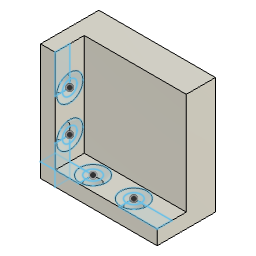
Step3-CornerMagBox-16X (Autodesk Fusion 360 design; units mm, degrees)
Autodesk Fusion 360 part; units mm, degrees
note: some values were not read from the file. Set by a fixed rule: which sketch regions a step uses.
sketch "Sketch1" plane through (0, 0, 0) normal (0, 1, 0) x (1, 0, 0)
  line L0 (0, 0) -> (40, 0)
  line L1 (40, 0) -> (40, -40)
  line L2 (40, -40) -> (0, -40)
  line L3 (0, -40) -> (0, 0)
  dimension "d1" = 40
  dimension "d2" = 40
  constraint horizontal L0
  constraint vertical L1
  constraint horizontal L2
  constraint vertical L3
  constraint coincident L0.start L3.end
  measures "d1" distance of L0.start L0.end
  measures "d2" distance of L0.start L2.end
extrude "Extrude1" add sketch "Sketch1" along normal blind 20
ref_plane "WorkPlane1" through (20, 0, 20) normal (0, -1, 0) x (-1, 0, 0)
sketch "Sketch2" plane through (20, 0, 20) normal (0, -1, 0) x (1, 0, 0)
  line L0 (20, 20) -> (-15, 20)
  line L1 (-15, 20) -> (-15, -15)
  line L2 (-15, -15) -> (20, -15)
  line L3 (20, -15) -> (20, 20)
  dimension "d6" = 35
  dimension "d7" = 35
  constraint horizontal L0
  constraint vertical L1
  constraint horizontal L2
  constraint vertical L3
  measures "d6" distance of L0.start L0.end
  measures "d7" distance of L0.start L2.end
extrude "Extrude2" cut sketch "Sketch2" against normal blind 10
ref_plane "WorkPlane2" through (5, 5, 22.5) normal (1, 0, 0) x (0, 0, -1)
sketch "Sketch3" plane through (5, 5, 22.5) normal (1, 0, 0) x (0, 1, 0)
  circle A0 centre (0, 4.5) radius 2.5
  circle A1 centre (0, -9.5) radius 2.5
  line L0 (-5, 17.5) -> (0, 17.5)
  line L1 (0, 17.5) -> (0, 4.5)
  line L2 (0, 4.5) -> (-5, 4.5)
  line L3 (-5, 4.5) -> (-5, 17.5)
  line L4 (-5, -22.5) -> (0, -22.5)
  line L5 (0, -22.5) -> (0, -9.5)
  line L6 (0, -9.5) -> (-5, -9.5)
  line L7 (-5, -9.5) -> (-5, -22.5)
  circle A2 centre (0, 4.5) radius 4.5
  circle A3 centre (0, -9.5) radius 4.5
  dimension "d11" = 5
  dimension "d12" = 5
  dimension "d35" = 5
  dimension "d36" = 13
  dimension "d37" = 5
  dimension "d38" = 13
  dimension "d39" = 9
  dimension "d40" = 9
  constraint horizontal L0
  constraint vertical L1
  constraint horizontal L2
  constraint vertical L3
  constraint horizontal L4
  constraint vertical L5
  constraint horizontal L6
  constraint vertical L7
  constraint coincident A0.centre L1.end
  constraint coincident A1.centre L5.end
  constraint concentric A0 A2
  constraint concentric A1 A3
  measures "d11" diameter of A0
  measures "d12" diameter of A1
  measures "d35" distance of L0.start L0.end
  measures "d36" distance of L0.start L2.end
  measures "d37" distance of L4.start L4.end
  measures "d38" distance of L4.start L6.end
  measures "d39" diameter of A2
  measures "d40" diameter of A3
extrude "Extrude7" cut sketch "Sketch3" against normal blind 2.5 draft -40 contours A0 L1 L2 | A0 L1 L2 A2 | A0 L1 L2 | A0 L1 L2 A2 | A1 L5 L6 | A1 L5 L6 A3 | A1 L5 L6 | A1 L5 L6 A3
extrude "Extrude3" cut sketch "Sketch3" against normal blind 10 contours A0 L1 L2 | A0 L1 L2 | A1 L5 L6 | A1 L5 L6
ref_plane "WorkPlane3" through (22.5, 5, 5) normal (0, 0, 1) x (1, 0, 0)
sketch "Sketch4" plane through (22.5, 5, 5) normal (0, 0, 1) x (1, 0, 0)
  circle A0 centre (-9.5, 0) radius 2.5
  circle A1 centre (4.5, 0) radius 2.5
  line L0 (-22.5, -5) -> (-9.5, -5)
  line L1 (-9.5, -5) -> (-9.5, 0)
  line L2 (-9.5, 0) -> (-22.5, 0)
  line L3 (-22.5, 0) -> (-22.5, -5)
  line L4 (17.5, -5) -> (4.5, -5)
  line L5 (4.5, -5) -> (4.5, 0)
  line L6 (4.5, 0) -> (17.5, 0)
  line L7 (17.5, 0) -> (17.5, -5)
  circle A2 centre (-9.5, 0) radius 4.5
  circle A3 centre (4.5, 0) radius 4.5
  dimension "d16" = 5
  dimension "d17" = 5
  dimension "d27" = 13
  dimension "d28" = 5
  dimension "d29" = 13
  dimension "d30" = 5
  dimension "d31" = 9
  dimension "d32" = 9
  constraint horizontal L0
  constraint vertical L1
  constraint horizontal L2
  constraint vertical L3
  constraint coincident A0.centre L1.end
  constraint horizontal L4
  constraint vertical L5
  constraint horizontal L6
  constraint vertical L7
  constraint coincident A1.centre L5.end
  constraint concentric A0 A2
  constraint concentric A1 A3
  measures "d16" diameter of A0
  measures "d17" diameter of A1
  measures "d27" distance of L0.start L0.end
  measures "d28" distance of L0.start L2.end
  measures "d29" distance of L4.start L4.end
  measures "d30" distance of L4.start L6.end
  measures "d31" diameter of A2
  measures "d32" diameter of A3
extrude "Extrude6" cut sketch "Sketch4" against normal blind 2.5 draft -40 contours A0 L1 L2 | A0 L1 L2 A2 | A0 L1 L2 | A0 L1 L2 A2 | A1 L5 L6 | A1 L5 L6 A3 | A1 L5 L6 | A1 L5 L6 A3
extrude "Extrude4" cut sketch "Sketch4" against normal blind 10 contours A0 L1 L2 | A0 L1 L2 | A1 L5 L6 | A1 L5 L6
ref_plane "WorkPlane4" through (22.5, 10, 22.5) normal (0, -1, 0) x (0, 0, -1)
sketch "Sketch5" plane through (22.5, 10, 22.5) normal (0, -1, 0) x (1, 0, 0)
ref_plane "WorkPlane5" through (20, 20, 20) normal (0, 1, 0) x (0, 0, 1)
sketch "Sketch6" plane through (20, 20, 20) normal (0, 1, 0) x (1, 0, 0)
  line L0 (-20, -20) -> (0, -20)
  line L1 (0, -20) -> (0, 0)
  line L2 (0, 0) -> (-20, 0)
  line L3 (-20, 0) -> (-20, -20)
  circle A0 centre (0, 0) radius 7.5
  dimension "d22" = 20
  dimension "d23" = 20
  dimension "d24" = 15
  constraint horizontal L0
  constraint vertical L1
  constraint horizontal L2
  constraint vertical L3
  constraint coincident L1.end L2.start
  measures "d22" distance of L0.start L0.end
  measures "d23" distance of L0.start L2.end
  measures "d24" diameter of A0
extrude "Extrude5" cut sketch "Sketch6" against normal blind 2.65 contours L1 L2 A0 | L1 L2 A0
